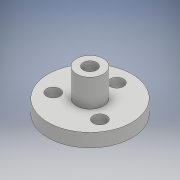
# Autodesk Inventor part: Part1
Saved by Autodesk Inventor 2018 (Build 220112000, 112)
## iProperties
Created: 2017-11-09
Part Number: Part1
Material: Generic
Document SubType Name: Modeling
Designer: kurtis
Density: 1 g/cm^3
Appearance: Default
Author: kurtis
Autodesk Inventor part; units mm, degrees
ref_plane "YZ Plane" through (0, 0, 0) normal (1, 0, 0) x (0, 1, 0)
ref_plane "XZ Plane" through (0, 0, 0) normal (0, 1, 0) x (-1, 0, 0)
ref_plane "XY Plane" through (0, 0, 0) normal (0, 0, 1) x (1, 0, 0)
sketch "Sketch1" plane through (0, 0, 0) normal (0, 0, 1) x (1, 0, 0)
  circle A0 centre (0, 0) radius 13.25
  circle A1 centre (0, 8.5) radius 2.125
  circle A2 centre (0, 0) radius 2.125
  circle A3 centre (0, 0) radius 4.25
  circle A4 centre (-7.3612, -4.25) radius 2.125
  circle A5 centre (7.3612, -4.25) radius 2.125
  dimension "d0" = 26.5
  dimension "d1" = 4.25
  dimension "d2" = 8.5
  dimension "d3" = 0
  dimension "d4" = 4.25
  dimension "d5" = 8.5
  dimension "d8" = 360
  constraints: 6 centre point, 3 coincident, 7 other
  measures "d0" diameter of A0
  measures "d1" diameter of A1
  measures "d2" distance of point (0, 0) A1.centre
  measures "d3" horizontal distance of A1.centre point (0, 0)
  measures "d4" diameter of A2
  measures "d5" diameter of A3
extrude "Extrusion1" add sketch "Sketch1" along normal blind 4.25 contours A0 | A3
extrude "Extrusion2" add sketch "Sketch1" along normal blind 13 contours A3
equation "\"d4\" = d1"
equation "\"d5\" = 2 * d1"
equation "\"d10\" = d1"
body "Solid1"
